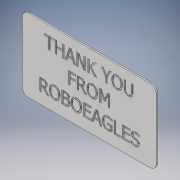
# Autodesk Inventor part: campbellPlacard
Saved by Autodesk Inventor 2017 (Build 210142000, 142)
## iProperties
Created: 2017-04-11
Part Number: campbellPlacard
Material: Generic
Document SubType Name: Sheet Metal
Designer: admin
Density: 1 g/cm^3
Sheet Metal Rule: Default
Appearance: Default
Author: admin
Autodesk Inventor part; units mm, degrees
ref_plane "YZ Plane" through (0, 0, 0) normal (1, 0, 0) x (0, 1, 0)
ref_plane "XZ Plane" through (0, 0, 0) normal (0, 1, 0) x (-1, 0, 0)
ref_plane "XY Plane" through (0, 0, 0) normal (0, 0, 1) x (1, 0, 0)
sketch "Sketch1" plane through (0, 0, 0) normal (0, 0, 1) x (1, 0, 0)
  line L0 (12.7, 0) -> (266.7, 0)
  line L1 (279.4, 12.7) -> (279.4, 139.7)
  line L2 (266.7, 152.4) -> (12.7, 152.4)
  line L3 (0, 139.7) -> (0, 12.7)
  arc A0 (12.7, 152.4) -> (0, 139.7) centre (12.7, 139.7) ccw
  arc A1 (279.4, 139.7) -> (266.7, 152.4) centre (266.7, 139.7) ccw
  arc A2 (266.7, 0) -> (279.4, 12.7) centre (266.7, 12.7) ccw
  arc A3 (0, 12.7) -> (12.7, 0) centre (12.7, 12.7) ccw
  point P0 (0, 0)
  point P1 (279.4, 152.4)
  point P2 (0, 152.4)
  dimension "d0" = 0
  dimension "d1" = 0
  dimension "d2" = 279.4
  dimension "d3" = 152.4
  dimension "d4" = 279.4
  dimension "d5" = 12.7
  measures "d0" distance from line of point (0, 0) L3
  measures "d1" distance from line of L0 point (0, 0)
  measures "d2" distance of point (279.4, 152.4) point (0, 152.4)
  measures "d3" distance between parallel lines of L2 L0
  measures "d4" distance between parallel lines of L3 L1
  measures "d5" radius of A0
extrude "Plate1" add sketch "Sketch1" along normal blind 3.175
sketch "Sketch2" plane through (0, 0, 3.175) normal (0, 0, 1) x (1, 0, 0)
  line L0 (12.7, 152.4) -> (266.7, 152.4) projected
  arc A0 (12.7, 152.4) -> (0, 139.7) centre (12.7, 139.7) ccw projected
  line L1 (0, 12.7) -> (0, 139.7) projected
  arc A1 (0, 12.7) -> (12.7, 0) centre (12.7, 12.7) ccw projected
  line L2 (266.7, 0) -> (12.7, 0) projected
  arc A2 (266.7, 0) -> (279.4, 12.7) centre (266.7, 12.7) ccw projected
  line L3 (279.4, 139.7) -> (279.4, 12.7) projected
  arc A3 (279.4, 139.7) -> (266.7, 152.4) centre (266.7, 139.7) ccw projected
  line L4 (12.7, 152.4) -> (266.7, 152.4) projected
  line L5 (279.4, 139.7) -> (279.4, 12.7) projected
  line L6 (31.75, 133.35) -> (247.65, 133.35) construction
  line L7 (247.65, 133.35) -> (247.65, 19.05) construction
  line L8 (247.65, 19.05) -> (31.75, 19.05) construction
  line L9 (31.75, 19.05) -> (31.75, 133.35) construction
  line L10 (54.4639, 107.4148) -> (54.4639, 129.8096)
  line L11 (54.4639, 129.8096) -> (45.9423, 129.8096)
  line L12 (45.9423, 129.8096) -> (45.9423, 132.8148)
  line L13 (45.9423, 132.8148) -> (66.3611, 132.8148)
  line L14 (66.3611, 132.8148) -> (66.3611, 129.8096)
  line L15 (66.3611, 129.8096) -> (57.8395, 129.8096)
  line L16 (57.8395, 129.8096) -> (57.8395, 107.4148)
  line L17 (57.8395, 107.4148) -> (54.4639, 107.4148)
  line L18 (87.3768, 107.4148) -> (84.0011, 107.4148)
  line L19 (84.0011, 107.4148) -> (84.0011, 119.8472)
  line L20 (84.0011, 119.8472) -> (72.3097, 119.8472)
  line L21 (72.3097, 119.8472) -> (72.3097, 107.4148)
  line L22 (72.3097, 107.4148) -> (68.934, 107.4148)
  line L23 (68.934, 107.4148) -> (68.934, 132.8148)
  line L24 (68.934, 132.8148) -> (72.3097, 132.8148)
  line L25 (72.3097, 132.8148) -> (72.3097, 122.8524)
  line L26 (72.3097, 122.8524) -> (84.0011, 122.8524)
  line L27 (84.0011, 122.8524) -> (84.0011, 132.8148)
  line L28 (84.0011, 132.8148) -> (87.3768, 132.8148)
  line L29 (87.3768, 132.8148) -> (87.3768, 107.4148)
  line L30 (89.7851, 107.4148) -> (98.3478, 132.8148)
  line L31 (98.3478, 132.8148) -> (102.5057, 132.8148)
  line L32 (102.5057, 132.8148) -> (111.0684, 107.4148)
  line L33 (111.0684, 107.4148) -> (107.5075, 107.4148)
  line L34 (107.5075, 107.4148) -> (105.2021, 114.5161)
  line L35 (105.2021, 114.5161) -> (95.5073, 114.5161)
  line L36 (95.5073, 114.5161) -> (93.2019, 107.4148)
  line L37 (93.2019, 107.4148) -> (89.7851, 107.4148)
  line L38 (104.2758, 117.3978) -> (100.3444, 129.3568)
  line L39 (100.3444, 129.3568) -> (96.4335, 117.3978)
  line L40 (96.4335, 117.3978) -> (104.2758, 117.3978)
  line L41 (131.6519, 107.4148) -> (127.8645, 107.4148)
  line L42 (127.8645, 107.4148) -> (116.6259, 129.3156)
  line L43 (116.6259, 129.3156) -> (116.6259, 107.4148)
  line L44 (116.6259, 107.4148) -> (113.4767, 107.4148)
  line L45 (113.4767, 107.4148) -> (113.4767, 132.8148)
  line L46 (113.4767, 132.8148) -> (118.2726, 132.8148)
  line L47 (118.2726, 132.8148) -> (128.5026, 112.7048)
  line L48 (128.5026, 112.7048) -> (128.5026, 132.8148)
  line L49 (128.5026, 132.8148) -> (131.6519, 132.8148)
  line L50 (131.6519, 132.8148) -> (131.6519, 107.4148)
  line L51 (155.3229, 107.4148) -> (150.9386, 107.4148)
  line L52 (150.9386, 107.4148) -> (141.6554, 119.2297)
  line L53 (141.6554, 119.2297) -> (140.1734, 117.5625)
  line L54 (140.1734, 117.5625) -> (140.1734, 107.4148)
  line L55 (140.1734, 107.4148) -> (136.7977, 107.4148)
  line L56 (136.7977, 107.4148) -> (136.7977, 132.8148)
  line L57 (136.7977, 132.8148) -> (140.1734, 132.8148)
  line L58 (140.1734, 132.8148) -> (140.1734, 121.144)
  line L59 (140.1734, 121.144) -> (150.5887, 132.8148)
  line L60 (150.5887, 132.8148) -> (154.7053, 132.8148)
  line L61 (154.7053, 132.8148) -> (144.1872, 121.4733)
  line L62 (144.1872, 121.4733) -> (155.3229, 107.4148)
  line L63 (186.0334, 132.8148) -> (177.4501, 118.6534)
  line L64 (177.4501, 118.6534) -> (177.4501, 107.4148)
  line L65 (177.4501, 107.4148) -> (174.0744, 107.4148)
  line L66 (174.0744, 107.4148) -> (174.0744, 118.3035)
  line L67 (174.0744, 118.3035) -> (165.4911, 132.8148)
  line L68 (165.4911, 132.8148) -> (169.2373, 132.8148)
  line L69 (169.2373, 132.8148) -> (175.7828, 121.638)
  line L70 (175.7828, 121.638) -> (182.4519, 132.8148)
  line L71 (182.4519, 132.8148) -> (186.0334, 132.8148)
  spline S0 degree 2 poles (206.3493, 129.9126) (207.7901, 128.2247) (209.3956, 123.2847) (209.3956, 120.1148) knots 0 0 0 1 2 2 2
  spline S1 degree 2 poles (209.3956, 120.1148) (209.3956, 117.0273) (207.8313, 112.0255) (206.3493, 110.3377) knots 0 0 0 1 2 2 2
  spline S2 degree 2 poles (206.3493, 110.3377) (204.7849, 108.5675) (200.6476, 106.8797) (198.157, 106.8797) knots 0 0 0 1 2 2 2
  spline S3 degree 2 poles (198.157, 106.8797) (195.5841, 106.8797) (191.4674, 108.6293) (189.9648, 110.3377) knots 0 0 0 1 2 2 2
  spline S4 degree 2 poles (189.9648, 110.3377) (188.5034, 112.0255) (186.9391, 116.9861) (186.9391, 120.1148) knots 0 0 0 1 2 2 2
  spline S5 degree 2 poles (186.9391, 120.1148) (186.9391, 123.3053) (188.524, 128.163) (189.9854, 129.9126) knots 0 0 0 1 2 2 2
  spline S6 degree 2 poles (189.9854, 129.9126) (191.4674, 131.6004) (195.6047, 133.35) (198.157, 133.35) knots 0 0 0 1 2 2 2
  spline S7 degree 2 poles (198.157, 133.35) (200.7506, 133.35) (204.9084, 131.5387) (206.3493, 129.9126) knots 0 0 0 1 2 2 2
  spline S8 degree 2 poles (205.8758, 120.1148) (205.8758, 122.626) (204.7849, 126.5163) (203.7969, 127.7925) knots 0 0 0 1 2 2 2
  spline S9 degree 2 poles (203.7969, 127.7925) (202.7883, 129.1098) (199.9478, 130.4271) (198.1776, 130.4271) knots 0 0 0 1 2 2 2
  spline S10 degree 2 poles (198.1776, 130.4271) (196.3457, 130.4271) (193.5875, 129.151) (192.5378, 127.7925) knots 0 0 0 1 2 2 2
  spline S11 degree 2 poles (192.5378, 127.7925) (191.5292, 126.4957) (190.4588, 122.5848) (190.4588, 120.1148) knots 0 0 0 1 2 2 2
  spline S12 degree 2 poles (190.4588, 120.1148) (190.4588, 115.113) (194.6579, 109.8025) (198.1776, 109.8025) knots 0 0 0 1 2 2 2
  spline S13 degree 2 poles (198.1776, 109.8025) (201.6974, 109.8025) (205.8758, 115.113) (205.8758, 120.1148) knots 0 0 0 1 2 2 2
  spline S14 degree 2 poles (221.9721, 106.8797) (219.7285, 106.8797) (216.394, 108.0529) (215.2207, 109.2262) knots 0 0 0 1 2 2 2
  spline S15 degree 2 poles (215.2207, 109.2262) (213.8828, 110.5435) (212.7919, 114.2485) (212.7919, 116.9656) knots 0 0 0 1 2 2 2
  line L72 (212.7919, 116.9656) -> (212.7919, 132.8148)
  line L73 (212.7919, 132.8148) -> (216.1676, 132.8148)
  line L74 (216.1676, 132.8148) -> (216.1676, 116.9656)
  spline S16 degree 2 poles (216.1676, 116.9656) (216.1676, 115.1954) (216.6204, 112.8077) (217.2585, 111.8403) knots 0 0 0 1 2 2 2
  spline S17 degree 2 poles (217.2585, 111.8403) (217.9378, 110.8111) (220.2843, 109.7613) (221.9721, 109.7613) knots 0 0 0 1 2 2 2
  spline S18 degree 2 poles (221.9721, 109.7613) (223.557, 109.7613) (226.0271, 110.8111) (226.7063, 111.8403) knots 0 0 0 1 2 2 2
  spline S19 degree 2 poles (226.7063, 111.8403) (227.3444, 112.8077) (227.7972, 115.1748) (227.7972, 116.8832) knots 0 0 0 1 2 2 2
  line L75 (227.7972, 116.8832) -> (227.7972, 132.8148)
  line L76 (227.7972, 132.8148) -> (231.1729, 132.8148)
  line L77 (231.1729, 132.8148) -> (231.1729, 116.9656)
  spline S20 degree 2 poles (231.1729, 116.9656) (231.1729, 114.3103) (230.1026, 110.5229) (228.7441, 109.2262) knots 0 0 0 1 2 2 2
  spline S21 degree 2 poles (228.7441, 109.2262) (227.5297, 108.0323) (224.3186, 106.8797) (221.9721, 106.8797) knots 0 0 0 1 2 2 2
  line L78 (111.6962, 87.9892) -> (99.8813, 87.9892)
  line L79 (99.8813, 87.9892) -> (99.8813, 80.8262)
  line L80 (99.8813, 80.8262) -> (111.2022, 80.8262)
  line L81 (111.2022, 80.8262) -> (111.2022, 77.821)
  line L82 (111.2022, 77.821) -> (99.8813, 77.821)
  line L83 (99.8813, 77.821) -> (99.8813, 65.5944)
  line L84 (99.8813, 65.5944) -> (96.5056, 65.5944)
  line L85 (96.5056, 65.5944) -> (96.5056, 90.9944)
  line L86 (96.5056, 90.9944) -> (111.6962, 90.9944)
  line L87 (111.6962, 90.9944) -> (111.6962, 87.9892)
  line L88 (134.3792, 65.5944) -> (129.9949, 65.5944)
  line L89 (129.9949, 65.5944) -> (121.9673, 75.7009)
  line L90 (121.9673, 75.7009) -> (118.0977, 75.7009)
  line L91 (118.0977, 75.7009) -> (118.0977, 65.5944)
  line L92 (118.0977, 65.5944) -> (114.722, 65.5944)
  line L93 (114.722, 65.5944) -> (114.722, 90.9944)
  line L94 (114.722, 90.9944) -> (121.2675, 90.9944)
  spline S22 degree 2 poles (121.2675, 90.9944) (123.4494, 90.9944) (126.3928, 90.521) (127.7307, 89.6565) knots 0 0 0 1 2 2 2
  spline S23 degree 2 poles (127.7307, 89.6565) (129.0686, 88.792) (130.6124, 86.0955) (130.6124, 84.0989) knots 0 0 0 1 2 2 2
  spline S24 degree 2 poles (130.6124, 84.0989) (130.6124, 81.3202) (127.7719, 77.5534) (125.343, 76.6477) knots 0 0 0 1 2 2 2
  line L95 (125.343, 76.6477) -> (134.3792, 65.5944)
  spline S25 degree 2 poles (127.0926, 83.8314) (127.0926, 84.9429) (126.3105, 86.6513) (125.4871, 87.207) knots 0 0 0 1 2 2 2
  spline S26 degree 2 poles (125.4871, 87.207) (124.7667, 87.6805) (122.8524, 88.0715) (121.4528, 88.0715) knots 0 0 0 1 2 2 2
  line L96 (121.4528, 88.0715) -> (118.0977, 88.0715)
  line L97 (118.0977, 88.0715) -> (118.0977, 78.5208)
  line L98 (118.0977, 78.5208) -> (121.0617, 78.5208)
  spline S27 degree 2 poles (121.0617, 78.5208) (122.5231, 78.5208) (124.849, 79.0354) (125.6518, 79.8382) knots 0 0 0 1 2 2 2
  spline S28 degree 2 poles (125.6518, 79.8382) (126.3928, 80.538) (127.0926, 82.514) (127.0926, 83.8314) knots 0 0 0 1 2 2 2
  spline S29 degree 2 poles (154.3657, 88.0921) (155.8066, 86.4043) (157.4121, 81.4643) (157.4121, 78.2944) knots 0 0 0 1 2 2 2
  spline S30 degree 2 poles (157.4121, 78.2944) (157.4121, 75.2069) (155.8477, 70.2051) (154.3657, 68.5173) knots 0 0 0 1 2 2 2
  spline S31 degree 2 poles (154.3657, 68.5173) (152.8014, 66.7471) (148.6641, 65.0592) (146.1735, 65.0592) knots 0 0 0 1 2 2 2
  spline S32 degree 2 poles (146.1735, 65.0592) (143.6006, 65.0592) (139.4839, 66.8088) (137.9813, 68.5173) knots 0 0 0 1 2 2 2
  spline S33 degree 2 poles (137.9813, 68.5173) (136.5199, 70.2051) (134.9555, 75.1657) (134.9555, 78.2944) knots 0 0 0 1 2 2 2
  spline S34 degree 2 poles (134.9555, 78.2944) (134.9555, 81.4848) (136.5404, 86.3425) (138.0019, 88.0921) knots 0 0 0 1 2 2 2
  spline S35 degree 2 poles (138.0019, 88.0921) (139.4839, 89.78) (143.6212, 91.5296) (146.1735, 91.5296) knots 0 0 0 1 2 2 2
  spline S36 degree 2 poles (146.1735, 91.5296) (148.767, 91.5296) (152.9249, 89.7182) (154.3657, 88.0921) knots 0 0 0 1 2 2 2
  spline S37 degree 2 poles (153.8923, 78.2944) (153.8923, 80.8056) (152.8014, 84.6959) (151.8134, 85.972) knots 0 0 0 1 2 2 2
  spline S38 degree 2 poles (151.8134, 85.972) (150.8048, 87.2894) (147.9643, 88.6067) (146.1941, 88.6067) knots 0 0 0 1 2 2 2
  spline S39 degree 2 poles (146.1941, 88.6067) (144.3622, 88.6067) (141.604, 87.3305) (140.5542, 85.972) knots 0 0 0 1 2 2 2
  spline S40 degree 2 poles (140.5542, 85.972) (139.5456, 84.6753) (138.4753, 80.7644) (138.4753, 78.2944) knots 0 0 0 1 2 2 2
  spline S41 degree 2 poles (138.4753, 78.2944) (138.4753, 73.2926) (142.6743, 67.9821) (146.1941, 67.9821) knots 0 0 0 1 2 2 2
  spline S42 degree 2 poles (146.1941, 67.9821) (149.7139, 67.9821) (153.8923, 73.2926) (153.8923, 78.2944) knots 0 0 0 1 2 2 2
  line L99 (182.8944, 65.5944) -> (179.5187, 65.5944)
  line L100 (179.5187, 65.5944) -> (179.5187, 87.4746)
  line L101 (179.5187, 87.4746) -> (172.8908, 72.5928)
  line L102 (172.8908, 72.5928) -> (170.8325, 72.5928)
  line L103 (170.8325, 72.5928) -> (164.2664, 87.4746)
  line L104 (164.2664, 87.4746) -> (164.2664, 65.5944)
  line L105 (164.2664, 65.5944) -> (161.1171, 65.5944)
  line L106 (161.1171, 65.5944) -> (161.1171, 90.9944)
  line L107 (161.1171, 90.9944) -> (165.7278, 90.9944)
  line L108 (165.7278, 90.9944) -> (172.0675, 76.8536)
  line L109 (172.0675, 76.8536) -> (178.2014, 90.9944)
  line L110 (178.2014, 90.9944) -> (182.8944, 90.9944)
  line L111 (182.8944, 90.9944) -> (182.8944, 65.5944)
  line L112 (55.9356, 23.774) -> (51.5513, 23.774)
  line L113 (51.5513, 23.774) -> (43.5237, 33.8805)
  line L114 (43.5237, 33.8805) -> (39.6541, 33.8805)
  line L115 (39.6541, 33.8805) -> (39.6541, 23.774)
  line L116 (39.6541, 23.774) -> (36.2784, 23.774)
  line L117 (36.2784, 23.774) -> (36.2784, 49.174)
  line L118 (36.2784, 49.174) -> (42.8239, 49.174)
  spline S43 degree 2 poles (42.8239, 49.174) (45.0058, 49.174) (47.9492, 48.7006) (49.2871, 47.836) knots 0 0 0 1 2 2 2
  spline S44 degree 2 poles (49.2871, 47.836) (50.625, 46.9715) (52.1688, 44.2751) (52.1688, 42.2785) knots 0 0 0 1 2 2 2
  spline S45 degree 2 poles (52.1688, 42.2785) (52.1688, 39.4997) (49.3283, 35.733) (46.8994, 34.8273) knots 0 0 0 1 2 2 2
  line L119 (46.8994, 34.8273) -> (55.9356, 23.774)
  spline S46 degree 2 poles (48.649, 42.0109) (48.649, 43.1224) (47.8669, 44.8309) (47.0435, 45.3866) knots 0 0 0 1 2 2 2
  spline S47 degree 2 poles (47.0435, 45.3866) (46.3231, 45.86) (44.4088, 46.2511) (43.0092, 46.2511) knots 0 0 0 1 2 2 2
  line L120 (43.0092, 46.2511) -> (39.6541, 46.2511)
  line L121 (39.6541, 46.2511) -> (39.6541, 36.7004)
  line L122 (39.6541, 36.7004) -> (42.6181, 36.7004)
  spline S48 degree 2 poles (42.6181, 36.7004) (44.0795, 36.7004) (46.4054, 37.215) (47.2082, 38.0177) knots 0 0 0 1 2 2 2
  spline S49 degree 2 poles (47.2082, 38.0177) (47.9492, 38.7176) (48.649, 40.6936) (48.649, 42.0109) knots 0 0 0 1 2 2 2
  spline S50 degree 2 poles (75.9221, 46.2717) (77.363, 44.5839) (78.9685, 39.6438) (78.9685, 36.474) knots 0 0 0 1 2 2 2
  spline S51 degree 2 poles (78.9685, 36.474) (78.9685, 33.3864) (77.4041, 28.3847) (75.9221, 26.6968) knots 0 0 0 1 2 2 2
  spline S52 degree 2 poles (75.9221, 26.6968) (74.3578, 24.9266) (70.2205, 23.2388) (67.7299, 23.2388) knots 0 0 0 1 2 2 2
  spline S53 degree 2 poles (67.7299, 23.2388) (65.157, 23.2388) (61.0403, 24.9884) (59.5377, 26.6968) knots 0 0 0 1 2 2 2
  spline S54 degree 2 poles (59.5377, 26.6968) (58.0763, 28.3847) (56.5119, 33.3453) (56.5119, 36.474) knots 0 0 0 1 2 2 2
  spline S55 degree 2 poles (56.5119, 36.474) (56.5119, 39.6644) (58.0968, 44.5221) (59.5583, 46.2717) knots 0 0 0 1 2 2 2
  spline S56 degree 2 poles (59.5583, 46.2717) (61.0403, 47.9595) (65.1776, 49.7091) (67.7299, 49.7091) knots 0 0 0 1 2 2 2
  spline S57 degree 2 poles (67.7299, 49.7091) (70.3234, 49.7091) (74.4813, 47.8978) (75.9221, 46.2717) knots 0 0 0 1 2 2 2
  spline S58 degree 2 poles (75.4487, 36.474) (75.4487, 38.9852) (74.3578, 42.8754) (73.3698, 44.1516) knots 0 0 0 1 2 2 2
  spline S59 degree 2 poles (73.3698, 44.1516) (72.3612, 45.4689) (69.5207, 46.7863) (67.7505, 46.7863) knots 0 0 0 1 2 2 2
  spline S60 degree 2 poles (67.7505, 46.7863) (65.9186, 46.7863) (63.1604, 45.5101) (62.1106, 44.1516) knots 0 0 0 1 2 2 2
  spline S61 degree 2 poles (62.1106, 44.1516) (61.102, 42.8548) (60.0317, 38.944) (60.0317, 36.474) knots 0 0 0 1 2 2 2
  spline S62 degree 2 poles (60.0317, 36.474) (60.0317, 31.4722) (64.2307, 26.1617) (67.7505, 26.1617) knots 0 0 0 1 2 2 2
  spline S63 degree 2 poles (67.7505, 26.1617) (71.2703, 26.1617) (75.4487, 31.4722) (75.4487, 36.474) knots 0 0 0 1 2 2 2
  spline S64 degree 2 poles (99.9019, 31.5751) (99.9019, 29.6814) (98.461, 26.7792) (97.2672, 25.8323) knots 0 0 0 1 2 2 2
  spline S65 degree 2 poles (97.2672, 25.8323) (95.8263, 24.7208) (92.5536, 23.774) (89.9601, 23.774) knots 0 0 0 1 2 2 2
  line L123 (89.9601, 23.774) -> (82.6735, 23.774)
  line L124 (82.6735, 23.774) -> (82.6735, 49.174)
  line L125 (82.6735, 49.174) -> (89.4043, 49.174)
  spline S66 degree 2 poles (89.4043, 49.174) (92.1213, 49.174) (94.8383, 48.8241) (96.0733, 48.1448) knots 0 0 0 1 2 2 2
  spline S67 degree 2 poles (96.0733, 48.1448) (97.4524, 47.4244) (98.708, 45.0573) (98.708, 43.4518) knots 0 0 0 1 2 2 2
  spline S68 degree 2 poles (98.708, 43.4518) (98.708, 41.661) (96.8143, 38.8205) (95.1471, 38.0177) knots 0 0 0 1 2 2 2
  line L126 (95.1471, 38.0177) -> (95.1471, 37.8942)
  spline S69 degree 2 poles (95.1471, 37.8942) (97.4113, 37.2767) (99.9019, 34.004) (99.9019, 31.5751) knots 0 0 0 1 2 2 2
  spline S70 degree 2 poles (96.3821, 31.431) (96.3821, 32.8719) (95.5588, 34.7244) (94.3237, 35.383) knots 0 0 0 1 2 2 2
  spline S71 degree 2 poles (94.3237, 35.383) (93.521, 35.7947) (91.6273, 36.0417) (89.8777, 36.0417) knots 0 0 0 1 2 2 2
  line L127 (89.8777, 36.0417) -> (86.0492, 36.0417)
  line L128 (86.0492, 36.0417) -> (86.0492, 26.6557)
  line L129 (86.0492, 26.6557) -> (88.7868, 26.6557)
  spline S72 degree 2 poles (88.7868, 26.6557) (91.0098, 26.6557) (93.5622, 27.0673) (94.5502, 27.726) knots 0 0 0 1 2 2 2
  spline S73 degree 2 poles (94.5502, 27.726) (95.497, 28.4053) (96.3821, 30.0931) (96.3821, 31.431) knots 0 0 0 1 2 2 2
  spline S74 degree 2 poles (95.1883, 42.9783) (95.1883, 43.884) (94.5707, 45.2425) (93.8915, 45.6336) knots 0 0 0 1 2 2 2
  spline S75 degree 2 poles (93.8915, 45.6336) (93.0682, 46.0864) (91.0716, 46.2923) (89.2808, 46.2923) knots 0 0 0 1 2 2 2
  line L130 (89.2808, 46.2923) -> (86.0492, 46.2923)
  line L131 (86.0492, 46.2923) -> (86.0492, 38.8617)
  line L132 (86.0492, 38.8617) -> (89.8777, 38.8617)
  spline S76 degree 2 poles (89.8777, 38.8617) (91.4626, 38.8617) (92.9652, 39.191) (93.768, 39.7056) knots 0 0 0 1 2 2 2
  spline S77 degree 2 poles (93.768, 39.7056) (94.5502, 40.1996) (95.1883, 41.7845) (95.1883, 42.9783) knots 0 0 0 1 2 2 2
  spline S78 degree 2 poles (121.2263, 46.2717) (122.6672, 44.5839) (124.2727, 39.6438) (124.2727, 36.474) knots 0 0 0 1 2 2 2
  spline S79 degree 2 poles (124.2727, 36.474) (124.2727, 33.3864) (122.7083, 28.3847) (121.2263, 26.6968) knots 0 0 0 1 2 2 2
  spline S80 degree 2 poles (121.2263, 26.6968) (119.662, 24.9266) (115.5247, 23.2388) (113.0341, 23.2388) knots 0 0 0 1 2 2 2
  spline S81 degree 2 poles (113.0341, 23.2388) (110.4612, 23.2388) (106.3445, 24.9884) (104.8419, 26.6968) knots 0 0 0 1 2 2 2
  spline S82 degree 2 poles (104.8419, 26.6968) (103.3805, 28.3847) (101.8161, 33.3453) (101.8161, 36.474) knots 0 0 0 1 2 2 2
  spline S83 degree 2 poles (101.8161, 36.474) (101.8161, 39.6644) (103.4011, 44.5221) (104.8625, 46.2717) knots 0 0 0 1 2 2 2
  spline S84 degree 2 poles (104.8625, 46.2717) (106.3445, 47.9595) (110.4818, 49.7091) (113.0341, 49.7091) knots 0 0 0 1 2 2 2
  spline S85 degree 2 poles (113.0341, 49.7091) (115.6276, 49.7091) (119.7855, 47.8978) (121.2263, 46.2717) knots 0 0 0 1 2 2 2
  spline S86 degree 2 poles (120.7529, 36.474) (120.7529, 38.9852) (119.662, 42.8754) (118.674, 44.1516) knots 0 0 0 1 2 2 2
  spline S87 degree 2 poles (118.674, 44.1516) (117.6654, 45.4689) (114.8249, 46.7863) (113.0547, 46.7863) knots 0 0 0 1 2 2 2
  spline S88 degree 2 poles (113.0547, 46.7863) (111.2228, 46.7863) (108.4646, 45.5101) (107.4148, 44.1516) knots 0 0 0 1 2 2 2
  spline S89 degree 2 poles (107.4148, 44.1516) (106.4062, 42.8548) (105.3359, 38.944) (105.3359, 36.474) knots 0 0 0 1 2 2 2
  spline S90 degree 2 poles (105.3359, 36.474) (105.3359, 31.4722) (109.5349, 26.1617) (113.0547, 26.1617) knots 0 0 0 1 2 2 2
  spline S91 degree 2 poles (113.0547, 26.1617) (116.5745, 26.1617) (120.7529, 31.4722) (120.7529, 36.474) knots 0 0 0 1 2 2 2
  line L133 (127.9777, 23.774) -> (127.9777, 49.174)
  line L134 (127.9777, 49.174) -> (143.8682, 49.174)
  line L135 (143.8682, 49.174) -> (143.8682, 46.1688)
  line L136 (143.8682, 46.1688) -> (131.3534, 46.1688)
  line L137 (131.3534, 46.1688) -> (131.3534, 39.2116)
  line L138 (131.3534, 39.2116) -> (143.0242, 39.2116)
  line L139 (143.0242, 39.2116) -> (143.0242, 36.2064)
  line L140 (143.0242, 36.2064) -> (131.3534, 36.2064)
  line L141 (131.3534, 36.2064) -> (131.3534, 26.7792)
  line L142 (131.3534, 26.7792) -> (143.8682, 26.7792)
  line L143 (143.8682, 26.7792) -> (143.8682, 23.774)
  line L144 (143.8682, 23.774) -> (127.9777, 23.774)
  line L145 (144.8356, 23.774) -> (153.3983, 49.174)
  line L146 (153.3983, 49.174) -> (157.5562, 49.174)
  line L147 (157.5562, 49.174) -> (166.1189, 23.774)
  line L148 (166.1189, 23.774) -> (162.5579, 23.774)
  line L149 (162.5579, 23.774) -> (160.2526, 30.8753)
  line L150 (160.2526, 30.8753) -> (150.5578, 30.8753)
  line L151 (150.5578, 30.8753) -> (148.2524, 23.774)
  line L152 (148.2524, 23.774) -> (144.8356, 23.774)
  line L153 (159.3263, 33.757) -> (155.3949, 45.7159)
  line L154 (155.3949, 45.7159) -> (151.484, 33.757)
  line L155 (151.484, 33.757) -> (159.3263, 33.757)
  spline S92 degree 2 poles (179.1688, 23.28) (176.4724, 23.28) (172.0058, 24.9266) (170.4002, 26.5939) knots 0 0 0 1 2 2 2
  spline S93 degree 2 poles (170.4002, 26.5939) (168.7947, 28.2817) (167.0863, 33.2629) (167.0863, 36.4946) knots 0 0 0 1 2 2 2
  spline S94 degree 2 poles (167.0863, 36.4946) (167.0863, 39.5615) (168.8153, 44.4192) (170.4208, 46.1482) knots 0 0 0 1 2 2 2
  spline S95 degree 2 poles (170.4208, 46.1482) (171.9646, 47.8155) (176.493, 49.6268) (179.1894, 49.6268) knots 0 0 0 1 2 2 2
  spline S96 degree 2 poles (179.1894, 49.6268) (180.4861, 49.6268) (182.8327, 49.2563) (183.903, 48.927) knots 0 0 0 1 2 2 2
  spline S97 degree 2 poles (183.903, 48.927) (184.7675, 48.68) (186.867, 47.7743) (187.5051, 47.445) knots 0 0 0 1 2 2 2
  line L156 (187.5051, 47.445) -> (187.5051, 43.3694)
  line L157 (187.5051, 43.3694) -> (187.2169, 43.3694)
  spline S98 degree 2 poles (187.2169, 43.3694) (186.5788, 43.9252) (185.2409, 44.9338) (184.0059, 45.5101) knots 0 0 0 1 2 2 2
  spline S99 degree 2 poles (184.0059, 45.5101) (182.9767, 46.0247) (180.3215, 46.704) (178.7983, 46.704) knots 0 0 0 1 2 2 2
  spline S100 degree 2 poles (178.7983, 46.704) (175.1344, 46.704) (170.6061, 41.1876) (170.6061, 36.5975) knots 0 0 0 1 2 2 2
  spline S101 degree 2 poles (170.6061, 36.5975) (170.6061, 34.0451) (171.7999, 30.2166) (172.932, 28.8993) knots 0 0 0 1 2 2 2
  spline S102 degree 2 poles (172.932, 28.8993) (174.0229, 27.5819) (177.1105, 26.2028) (179.0453, 26.2028) knots 0 0 0 1 2 2 2
  spline S103 degree 2 poles (179.0453, 26.2028) (180.4656, 26.2028) (183.3061, 26.6145) (184.2735, 27.0262) knots 0 0 0 1 2 2 2
  line L158 (184.2735, 27.0262) -> (184.2735, 33.5923)
  line L159 (184.2735, 33.5923) -> (178.3866, 33.5923)
  line L160 (178.3866, 33.5923) -> (178.3866, 36.5563)
  line L161 (178.3866, 36.5563) -> (187.608, 36.5563)
  line L162 (187.608, 36.5563) -> (187.608, 25.4618)
  spline S104 degree 2 poles (187.608, 25.4618) (186.9699, 25.1736) (184.7881, 24.2886) (183.8618, 24.021) knots 0 0 0 1 2 2 2
  spline S105 degree 2 poles (183.8618, 24.021) (182.6062, 23.6505) (180.5891, 23.28) (179.1688, 23.28) knots 0 0 0 1 2 2 2
  line L163 (206.5654, 23.774) -> (191.8482, 23.774)
  line L164 (191.8482, 23.774) -> (191.8482, 49.174)
  line L165 (191.8482, 49.174) -> (195.2239, 49.174)
  line L166 (195.2239, 49.174) -> (195.2239, 26.7792)
  line L167 (195.2239, 26.7792) -> (206.5654, 26.7792)
  line L168 (206.5654, 26.7792) -> (206.5654, 23.774)
  line L169 (209.2207, 23.774) -> (209.2207, 49.174)
  line L170 (209.2207, 49.174) -> (225.1111, 49.174)
  line L171 (225.1111, 49.174) -> (225.1111, 46.1688)
  line L172 (225.1111, 46.1688) -> (212.5964, 46.1688)
  line L173 (212.5964, 46.1688) -> (212.5964, 39.2116)
  line L174 (212.5964, 39.2116) -> (224.2672, 39.2116)
  line L175 (224.2672, 39.2116) -> (224.2672, 36.2064)
  line L176 (224.2672, 36.2064) -> (212.5964, 36.2064)
  line L177 (212.5964, 36.2064) -> (212.5964, 26.7792)
  line L178 (212.5964, 26.7792) -> (225.1111, 26.7792)
  line L179 (225.1111, 26.7792) -> (225.1111, 23.774)
  line L180 (225.1111, 23.774) -> (209.2207, 23.774)
  spline S106 degree 2 poles (235.8968, 23.3211) (233.1387, 23.3211) (229.269, 24.4738) (227.5605, 25.2971) knots 0 0 0 1 2 2 2
  line L181 (227.5605, 25.2971) -> (227.5605, 29.5373)
  line L182 (227.5605, 29.5373) -> (227.8075, 29.5373)
  spline S107 degree 2 poles (227.8075, 29.5373) (229.4748, 27.973) (233.6944, 26.244) (235.6498, 26.244) knots 0 0 0 1 2 2 2
  spline S108 degree 2 poles (235.6498, 26.244) (238.4492, 26.244) (241.3103, 28.5699) (241.3103, 30.4842) knots 0 0 0 1 2 2 2
  spline S109 degree 2 poles (241.3103, 30.4842) (241.3103, 32.0074) (239.8077, 33.901) (238.1816, 34.3745) knots 0 0 0 1 2 2 2
  spline S110 degree 2 poles (238.1816, 34.3745) (237.0083, 34.7038) (235.0529, 35.1566) (233.5915, 35.5271) knots 0 0 0 1 2 2 2
  spline S111 degree 2 poles (233.5915, 35.5271) (232.2741, 35.877) (230.1952, 36.9268) (229.3925, 37.7707) knots 0 0 0 1 2 2 2
  spline S112 degree 2 poles (229.3925, 37.7707) (228.6103, 38.6147) (227.7458, 40.8788) (227.7458, 42.3608) knots 0 0 0 1 2 2 2
  spline S113 degree 2 poles (227.7458, 42.3608) (227.7458, 45.4484) (232.5623, 49.6268) (236.2879, 49.6268) knots 0 0 0 1 2 2 2
  spline S114 degree 2 poles (236.2879, 49.6268) (238.4286, 49.6268) (242.216, 48.7829) (243.8421, 47.9801) knots 0 0 0 1 2 2 2
  line L183 (243.8421, 47.9801) -> (243.8421, 43.9458)
  line L184 (243.8421, 43.9458) -> (243.5951, 43.9458)
  spline S115 degree 2 poles (243.5951, 43.9458) (242.3806, 45.0573) (238.5933, 46.704) (236.5143, 46.704) knots 0 0 0 1 2 2 2
  spline S116 degree 2 poles (236.5143, 46.704) (234.1678, 46.704) (231.2656, 44.5015) (231.2656, 42.7108) knots 0 0 0 1 2 2 2
  spline S117 degree 2 poles (231.2656, 42.7108) (231.2656, 41.1053) (232.974, 39.191) (234.5795, 38.7587) knots 0 0 0 1 2 2 2
  spline S118 degree 2 poles (234.5795, 38.7587) (235.6498, 38.4706) (238.7579, 37.7296) (239.7871, 37.4208) knots 0 0 0 1 2 2 2
  spline S119 degree 2 poles (239.7871, 37.4208) (242.4012, 36.6181) (244.8301, 33.3864) (244.8301, 31.0194) knots 0 0 0 1 2 2 2
  spline S120 degree 2 poles (244.8301, 31.0194) (244.8301, 29.5168) (243.6156, 26.6351) (242.5247, 25.6265) knots 0 0 0 1 2 2 2
  spline S121 degree 2 poles (242.5247, 25.6265) (241.3103, 24.515) (238.2228, 23.3211) (235.8968, 23.3211) knots 0 0 0 1 2 2 2
  point P0 (0, 0)
  dimension "d7" = 215.9
  dimension "d8" = 114.3
  dimension "d9" = 19.05
  dimension "d10" = 31.75
  constraints: 2 other
  measures "d7" distance between parallel lines of L9 L7
  measures "d8" distance of L6.end L7.end
  measures "d9" distance between parallel lines of L0 L6
  measures "d10" distance between parallel lines of L1 L9
extrude "Extrusion1" cut sketch "Sketch2" against normal up to next contours L10 L11 L12 L13 L14 L15 L16 L17 | L18 L19 L20 L21 L22 L23 L24 L25 L26 L27 L28 L29 | L30 L31 L32 L33 L34 L35 L36 L37 | L41 L42 L43 L44 L45 L46 L47 L48 L49 L50 | L51 L52 L53 L54 L55 L56 L57 L58 L59 L60 L61 L62 | L63 L64 L65 L66 L67 L68 L69 L70 L71 | S0 S1 S2 S3 S4 S5 S6 S7 | S14 S15 L72 L73 L74 S16 S17 S18 S19 L75 L76 L77 S20 S21 | L78 L79 L80 L81 L82 L83 L84 L85 L86 L87 | L88 L89 L90 L91 L92 L93 L94 S22 S23 S24 L95 | S29 S30 S31 S32 S33 S34 S35 S36 | L99 L100 L101 L102 L103 L104 L105 L106 L107 L108 L109 L110 L111 | L112 L113 L114 L115 L116 L117 L118 S43 S44 S45 L119 | S50 S51 S52 S53 S54 S55 S56 S57 | S64 S65 L123 L124 L125 S66 S67 S68 L126 S69 | S78 S79 S80 S81 S82 S83 S84 S85 | L133 L134 L135 L136 L137 L138 L139 L140 L141 L142 L143 L144 | L145 L146 L147 L148 L149 L150 L151 L152 | S92 S93 S94 S95 S96 S97 L156 L157 S98 S99 S100 S101 S102 S103 L158 L159 L160 L161 L162 S104 S105 | L163 L164 L165 L166 L167 L168 | L169 L170 L171 L172 L173 L174 L175 L176 L177 L178 L179 L180 | S106 L181 L182 S107 S108 S109 S110 S111 S112 S113 S114 L183 L184 S115 S116 S117 S118 S119 S120 S121
equation "\"BendRadius\" = Thickness"
equation "\"BendReliefWidth\" = Thickness"
equation "\"BendReliefDepth\" = 0.5 * Thickness"
equation "\"CornerReliefSize\" = 4 * Thickness"
equation "\"MinimumRemnant\" = 2 * Thickness"
equation "\"TransitionRadius\" = BendRadius"
equation "\"JacobiRadiusSize\" = Thickness"
equation "\"GapSize\" = Thickness"
equation "\"d6\" = BendRadius"
equation "\"Thickness\" = 3.175"
body "Solid1"
